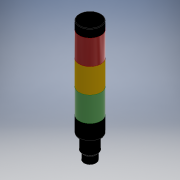
# Autodesk Inventor part: Light Stack
Saved by Autodesk Inventor 2017 (Build 210142000, 142)
## iProperties
Created: 2020-05-28
Part Number: Light Stack
Material: Generic
Document SubType Name: Modeling
Designer: Sid
Density: 1 g/cm^3
Appearance: Default
Author: Sid
Autodesk Inventor part; units mm, degrees
ref_plane "YZ Plane" through (0, 0, 0) normal (1, 0, 0) x (0, 1, 0)
ref_plane "XZ Plane" through (0, 0, 0) normal (0, 1, 0) x (-1, 0, 0)
ref_plane "XY Plane" through (0, 0, 0) normal (0, 0, 1) x (1, 0, 0)
sketch "Sketch1" plane through (0, 0, 0) normal (0, 0, 1) x (1, 0, 0)
  circle A0 centre (0, 0) radius 11
  dimension "d0" = 22
  constraints: 1 centre point, 1 coincident
  measures "d0" diameter of A0
extrude "Extrusion1" add sketch "Sketch1" along normal blind 16.6
sketch "Sketch2" plane through (0, 0, 16.6) normal (0, 0, 1) x (1, 0, 0)
  circle A0 centre (0, 0) radius 14
  dimension "d3" = 28
  constraints: 1 centre point, 1 coincident
  measures "d3" diameter of A0
extrude "Extrusion2" add sketch "Sketch2" along normal blind 25.4
sketch "Sketch3" plane through (0, 0, 0) normal (0, 0, -1) x (-1, 0, 0)
  circle A0 centre (0, 0) radius 9
  dimension "d6" = 18
  constraints: 1 centre point, 1 coincident
  measures "d6" diameter of A0
extrude "Extrusion3" cut sketch "Sketch3" against normal through all
fillet "Fillet1" radius 1 1 edges at (-11, 0, 0)
fillet "Fillet2" radius 3 1 edges at (-11, 0, 16.6)
sketch "Sketch4" plane through (0, 0, 42) normal (0, 0, 1) x (1, 0, 0)
  circle A0 centre (0, 0) radius 19.8
  dimension "d11" = 39.6
  constraints: 1 centre point, 1 coincident
  measures "d11" diameter of A0
extrude "Extrusion4" add sketch "Sketch4" along normal blind 30 separate body
sketch "Sketch5" plane through (0, 0, 72) normal (0, 0, 1) x (1, 0, 0)
  circle A0 centre (0, 0) radius 19.8
  constraints: 1 centre point, 1 coincident
extrude "Extrusion5" add sketch "Sketch5" along normal blind 45 separate body
sketch "Sketch6" plane through (0, 0, 117) normal (0, 0, 1) x (1, 0, 0)
  circle A0 centre (0, 0) radius 19.8
  constraints: 1 centre point, 1 coincident
extrude "Extrusion6" add sketch "Sketch6" along normal blind 45 separate body
sketch "Sketch7" plane through (0, 0, 162) normal (0, 0, 1) x (1, 0, 0)
  circle A0 centre (0, 0) radius 19.8
  constraints: 1 centre point, 1 coincident
extrude "Extrusion7" add sketch "Sketch7" along normal blind 45 separate body
sketch "Sketch8" plane through (0, 0, 207) normal (0, 0, 1) x (1, 0, 0)
  circle A0 centre (0, 0) radius 19.8
  constraints: 1 centre point, 1 coincident
extrude "Extrusion8" add sketch "Sketch8" along normal blind 15 separate body
fillet "Fillet3" radius 1 2 edges at (-13.9995, 0, 16.6) (-14, 0, 16.6)
fillet "Fillet4" radius 3 1 edges at (-19.8, 0, 42)
fillet "Fillet5" radius 1 1 edges at (-19.8, 0, 222)
body "Solid1"
body "Solid2"
body "Solid3"
body "Solid4"
body "Solid5"
body "Solid6"
